Autodesk Inventor part; units mm, degrees
(part 2 of 4)
  line L557 (-1.0373, -25.9013) -> (-0.4998, -25.9013)
  spline S119 degree 2 poles (-0.4998, -25.9013) (-0.366, -25.9013) (-0.366, -26.0351) knots 0 0 0 1 1 1
  line L558 (-0.4998, -25.9013) -> (-0.366, -25.9013) construction
  line L559 (-0.366, -25.9013) -> (-0.366, -26.0351) construction
  line L560 (-0.366, -26.0351) -> (-0.366, -27.6364)
  spline S120 degree 2 poles (-0.366, -27.6364) (-0.366, -27.7703) (-0.4998, -27.7703) knots 0 0 0 1 1 1
  line L561 (-0.366, -27.6364) -> (-0.366, -27.7703) construction
  line L562 (-0.366, -27.7703) -> (-0.4998, -27.7703) construction
  spline S121 degree 2 poles (-7.9758, -27.7703) (-8.1096, -27.7703) (-8.1096, -27.6364) knots 0 0 0 1 1 1
  line L563 (-7.9758, -27.7703) -> (-8.1096, -27.7703) construction
  line L564 (-8.1096, -27.7703) -> (-8.1096, -27.6364) construction
  line L565 (-8.1096, -27.6364) -> (-8.1096, -26.4365)
  spline S122 degree 2 poles (-8.1096, -26.4365) (-8.1096, -26.3273) (-8.2657, -26.1689) (-8.375, -26.1689) knots 0 0 0 1 2 2 2
  line L566 (-8.1096, -26.4365) -> (-8.1096, -26.3273) construction
  line L567 (-8.1096, -26.3273) -> (-8.2657, -26.1689) construction
  line L568 (-8.2657, -26.1689) -> (-8.375, -26.1689) construction
  spline S123 degree 2 poles (-8.908, -27.6364) (-8.908, -27.7703) (-9.0418, -27.7703) knots 0 0 0 1 1 1
  line L569 (-8.908, -27.6364) -> (-8.908, -27.7703) construction
  line L570 (-8.908, -27.7703) -> (-9.0418, -27.7703) construction
  spline S124 degree 2 poles (-9.0418, -27.7703) (-9.1756, -27.7703) (-9.1756, -27.6364) knots 0 0 0 1 1 1
  line L571 (-9.0418, -27.7703) -> (-9.1756, -27.7703) construction
  line L572 (-9.1756, -27.7703) -> (-9.1756, -27.6364) construction
  line L573 (-9.1756, -27.6364) -> (-9.1756, -26.0351)
  spline S125 degree 2 poles (-9.1756, -26.0351) (-9.1756, -25.9013) (-9.0418, -25.9013) knots 0 0 0 1 1 1
  line L574 (-9.1756, -26.0351) -> (-9.1756, -25.9013) construction
  line L575 (-9.1756, -25.9013) -> (-9.0418, -25.9013) construction
  line L576 (-9.0418, -25.9013) -> (-8.375, -25.9013)
  spline S126 degree 2 poles (-8.375, -25.9013) (-8.1542, -25.9013) (-7.8419, -26.2135) (-7.8419, -26.4343) knots 0 0 0 1 2 2 2
  line L577 (-8.375, -25.9013) -> (-8.1542, -25.9013) construction
  line L578 (-8.1542, -25.9013) -> (-7.8419, -26.2135) construction
  line L579 (-7.8419, -26.2135) -> (-7.8419, -26.4343) construction
  line L580 (-7.8419, -26.4343) -> (-7.8419, -27.6364)
  spline S127 degree 2 poles (-7.8419, -27.6364) (-7.8419, -27.7703) (-7.9758, -27.7703) knots 0 0 0 1 1 1
  line L581 (-7.8419, -27.6364) -> (-7.8419, -27.7703) construction
  line L582 (-7.8419, -27.7703) -> (-7.9758, -27.7703) construction
  spline S128 degree 2 poles (-10.2439, -27.5026) (-10.1347, -27.5026) (-9.9785, -27.3443) (-9.9785, -27.235) knots 0 0 0 1 2 2 2
  line L583 (-10.2439, -27.5026) -> (-10.1347, -27.5026) construction
  line L584 (-10.1347, -27.5026) -> (-9.9785, -27.3443) construction
  line L585 (-9.9785, -27.3443) -> (-9.9785, -27.235) construction
  spline S129 degree 2 poles (-10.5116, -26.1689) (-10.6209, -26.1689) (-10.777, -26.3273) (-10.777, -26.4365) knots 0 0 0 1 2 2 2
  line L586 (-10.5116, -26.1689) -> (-10.6209, -26.1689) construction
  line L587 (-10.6209, -26.1689) -> (-10.777, -26.3273) construction
  line L588 (-10.777, -26.3273) -> (-10.777, -26.4365) construction
  line L589 (-10.777, -26.4365) -> (-10.777, -27.235)
  spline S130 degree 2 poles (-10.777, -27.235) (-10.777, -27.3443) (-10.6209, -27.5026) (-10.5116, -27.5026) knots 0 0 0 1 2 2 2
  line L590 (-10.777, -27.235) -> (-10.777, -27.3443) construction
  line L591 (-10.777, -27.3443) -> (-10.6209, -27.5026) construction
  line L592 (-10.6209, -27.5026) -> (-10.5116, -27.5026) construction
  line L593 (-10.5116, -27.5026) -> (-10.2439, -27.5026)
  line L594 (-10.2439, -27.7703) -> (-10.5116, -27.7703)
  spline S131 degree 2 poles (-10.5116, -27.7703) (-10.7302, -27.7703) (-11.0446, -27.458) (-11.0446, -27.2372) knots 0 0 0 1 2 2 2
  line L595 (-10.5116, -27.7703) -> (-10.7302, -27.7703) construction
  line L596 (-10.7302, -27.7703) -> (-11.0446, -27.458) construction
  line L597 (-11.0446, -27.458) -> (-11.0446, -27.2372) construction
  line L598 (-11.0446, -27.2372) -> (-11.0446, -26.4343)
  spline S132 degree 2 poles (-11.0446, -26.4343) (-11.0446, -26.2135) (-10.7302, -25.9013) (-10.5116, -25.9013) knots 0 0 0 1 2 2 2
  line L599 (-11.0446, -26.4343) -> (-11.0446, -26.2135) construction
  line L600 (-11.0446, -26.2135) -> (-10.7302, -25.9013) construction
  line L601 (-10.7302, -25.9013) -> (-10.5116, -25.9013) construction
  line L602 (-10.5116, -25.9013) -> (-9.8447, -25.9013)
  spline S133 degree 2 poles (-9.8447, -25.9013) (-9.7109, -25.9013) (-9.7109, -26.0351) knots 0 0 0 1 1 1
  line L603 (-9.8447, -25.9013) -> (-9.7109, -25.9013) construction
  line L604 (-9.7109, -25.9013) -> (-9.7109, -26.0351) construction
  line L605 (-9.7109, -26.0351) -> (-9.7109, -27.2328)
  spline S134 degree 2 poles (-9.7109, -27.2328) (-9.7109, -27.4335) (-9.5236, -27.5138) knots 0 0 0 1 1 1
  line L606 (-9.7109, -27.2328) -> (-9.7109, -27.4335) construction
  line L607 (-9.7109, -27.4335) -> (-9.5236, -27.5138) construction
  spline S135 degree 2 poles (-9.5236, -27.5138) (-9.441, -27.5472) (-9.441, -27.632) knots 0 0 0 1 1 1
  line L608 (-9.5236, -27.5138) -> (-9.441, -27.5472) construction
  line L609 (-9.441, -27.5472) -> (-9.441, -27.632) construction
  spline S136 degree 2 poles (-9.441, -27.632) (-9.441, -27.6877) (-9.5169, -27.7725) (-9.5726, -27.7725) knots 0 0 0 1 2 2 2
  line L610 (-9.441, -27.632) -> (-9.441, -27.6877) construction
  line L611 (-9.441, -27.6877) -> (-9.5169, -27.7725) construction
  line L612 (-9.5169, -27.7725) -> (-9.5726, -27.7725) construction
  spline S137 degree 2 poles (-9.5726, -27.7725) (-9.6016, -27.7725) (-9.6306, -27.7591) knots 0 0 0 1 1 1
  line L613 (-9.5726, -27.7725) -> (-9.6016, -27.7725) construction
  line L614 (-9.6016, -27.7725) -> (-9.6306, -27.7591) construction
  spline S138 degree 2 poles (-9.6306, -27.7591) (-9.7644, -27.7011) (-9.847, -27.5941) knots 0 0 0 1 1 1
  line L615 (-9.6306, -27.7591) -> (-9.7644, -27.7011) construction
  line L616 (-9.7644, -27.7011) -> (-9.847, -27.5941) construction
  spline S139 degree 2 poles (-9.847, -27.5941) (-10.0075, -27.7703) (-10.2439, -27.7703) knots 0 0 0 1 1 1
  line L617 (-9.847, -27.5941) -> (-10.0075, -27.7703) construction
  line L618 (-10.0075, -27.7703) -> (-10.2439, -27.7703) construction
  spline S140 degree 2 poles (8.3441, 56.8614) (8.338, 56.6518) (8.3229, 56.2658) (8.3137, 56.1108) knots 0 0 0 1 2 2 2
  line L619 (8.3441, 56.8614) -> (8.338, 56.6518) construction
  line L620 (8.338, 56.6518) -> (8.3229, 56.2658) construction
  line L621 (8.3229, 56.2658) -> (8.3137, 56.1108) construction
  spline S141 degree 2 poles (8.3137, 56.1108) (8.2985, 55.7158) (8.2256, 55.1809) (8.1709, 55.0199) knots 0 0 0 1 2 2 2
  line L622 (8.3137, 56.1108) -> (8.2985, 55.7158) construction
  line L623 (8.2985, 55.7158) -> (8.2256, 55.1809) construction
  line L624 (8.2256, 55.1809) -> (8.1709, 55.0199) construction
  spline S142 degree 2 poles (8.1709, 55.0199) (8.1162, 54.8527) (7.9825, 54.6674) (7.8974, 54.5914) knots 0 0 0 1 2 2 2
  line L625 (8.1709, 55.0199) -> (8.1162, 54.8527) construction
  line L626 (8.1162, 54.8527) -> (7.9825, 54.6674) construction
  line L627 (7.9825, 54.6674) -> (7.8974, 54.5914) construction
  spline S143 degree 2 poles (7.8974, 54.5914) (7.8123, 54.5154) (7.6178, 54.4394) (7.4932, 54.4394) knots 0 0 0 1 2 2 2
  line L628 (7.8974, 54.5914) -> (7.8123, 54.5154) construction
  line L629 (7.8123, 54.5154) -> (7.6178, 54.4394) construction
  line L630 (7.6178, 54.4394) -> (7.4932, 54.4394) construction
  spline S144 degree 2 poles (7.4932, 54.4394) (7.4537, 54.4394) (7.3261, 54.4455) (7.3018, 54.4455) knots 0 0 0 1 2 2 2
  line L631 (7.4932, 54.4394) -> (7.4537, 54.4394) construction
  line L632 (7.4537, 54.4394) -> (7.3261, 54.4455) construction
  line L633 (7.3261, 54.4455) -> (7.3018, 54.4455) construction
  spline S145 degree 2 poles (7.3261, 54.8588) (7.3443, 54.8588) (7.3838, 54.8527) (7.4081, 54.8527) knots 0 0 0 1 2 2 2
  line L634 (7.3261, 54.8588) -> (7.3443, 54.8588) construction
  line L635 (7.3443, 54.8588) -> (7.3838, 54.8527) construction
  line L636 (7.3838, 54.8527) -> (7.4081, 54.8527) construction
  spline S146 degree 2 poles (7.4081, 54.8527) (7.4689, 54.8527) (7.5844, 54.8892) (7.63, 54.9348) knots 0 0 0 1 2 2 2
  line L637 (7.4081, 54.8527) -> (7.4689, 54.8527) construction
  line L638 (7.4689, 54.8527) -> (7.5844, 54.8892) construction
  line L639 (7.5844, 54.8892) -> (7.63, 54.9348) construction
  spline S147 degree 2 poles (7.63, 54.9348) (7.7546, 55.0594) (7.8701, 55.6763) (7.8944, 56.2324) knots 0 0 0 1 2 2 2
  line L640 (7.63, 54.9348) -> (7.7546, 55.0594) construction
  line L641 (7.7546, 55.0594) -> (7.8701, 55.6763) construction
  line L642 (7.8701, 55.6763) -> (7.8944, 56.2324) construction
  spline S148 degree 2 poles (7.8944, 56.2324) (7.9065, 56.439) (7.9248, 57.0012) (7.9308, 57.2595) knots 0 0 0 1 2 2 2
  line L643 (7.8944, 56.2324) -> (7.9065, 56.439) construction
  line L644 (7.9065, 56.439) -> (7.9248, 57.0012) construction
  line L645 (7.9248, 57.0012) -> (7.9308, 57.2595) construction
  spline S149 degree 2 poles (5.8674, 54.7737) (6.2321, 54.7737) (6.6332, 55.3116) (6.6332, 55.8525) knots 0 0 0 1 2 2 2
  line L646 (5.8674, 54.7737) -> (6.2321, 54.7737) construction
  line L647 (6.2321, 54.7737) -> (6.6332, 55.3116) construction
  line L648 (6.6332, 55.3116) -> (6.6332, 55.8525) construction
  spline S150 degree 2 poles (6.6332, 55.8525) (6.6332, 56.3995) (6.2351, 56.9313) (5.8674, 56.9313) knots 0 0 0 1 2 2 2
  line L649 (6.6332, 55.8525) -> (6.6332, 56.3995) construction
  line L650 (6.6332, 56.3995) -> (6.2351, 56.9313) construction
  line L651 (6.2351, 56.9313) -> (5.8674, 56.9313) construction
  spline S151 degree 2 poles (5.8674, 56.9313) (5.4997, 56.9313) (5.0986, 56.3995) (5.0986, 55.8525) knots 0 0 0 1 2 2 2
  line L652 (5.8674, 56.9313) -> (5.4997, 56.9313) construction
  line L653 (5.4997, 56.9313) -> (5.0986, 56.3995) construction
  line L654 (5.0986, 56.3995) -> (5.0986, 55.8525) construction
  spline S152 degree 2 poles (5.0986, 55.8525) (5.0986, 55.3207) (5.4997, 54.7737) (5.8674, 54.7737) knots 0 0 0 1 2 2 2
  line L655 (5.0986, 55.8525) -> (5.0986, 55.3207) construction
  line L656 (5.0986, 55.3207) -> (5.4997, 54.7737) construction
  line L657 (5.4997, 54.7737) -> (5.8674, 54.7737) construction
  spline S153 degree 2 poles (5.8674, 54.3665) (5.2809, 54.3665) (4.6093, 55.1657) (4.6093, 55.8525) knots 0 0 0 1 2 2 2
  line L658 (5.8674, 54.3665) -> (5.2809, 54.3665) construction
  line L659 (5.2809, 54.3665) -> (4.6093, 55.1657) construction
  line L660 (4.6093, 55.1657) -> (4.6093, 55.8525) construction
  spline S154 degree 2 poles (4.6093, 55.8525) (4.6093, 56.5575) (5.3022, 57.3385) (5.8674, 57.3385) knots 0 0 0 1 2 2 2
  line L661 (4.6093, 55.8525) -> (4.6093, 56.5575) construction
  line L662 (4.6093, 56.5575) -> (5.3022, 57.3385) construction
  line L663 (5.3022, 57.3385) -> (5.8674, 57.3385) construction
  spline S155 degree 2 poles (5.8674, 57.3385) (6.4387, 57.3385) (7.1225, 56.5606) (7.1225, 55.8525) knots 0 0 0 1 2 2 2
  line L664 (5.8674, 57.3385) -> (6.4387, 57.3385) construction
  line L665 (6.4387, 57.3385) -> (7.1225, 56.5606) construction
  line L666 (7.1225, 56.5606) -> (7.1225, 55.8525) construction
  spline S156 degree 2 poles (7.1225, 55.8525) (7.1225, 55.1414) (6.4387, 54.3665) (5.8674, 54.3665) knots 0 0 0 1 2 2 2
  line L667 (7.1225, 55.8525) -> (7.1225, 55.1414) construction
  line L668 (7.1225, 55.1414) -> (6.4387, 54.3665) construction
  line L669 (6.4387, 54.3665) -> (5.8674, 54.3665) construction
  spline S157 degree 2 poles (3.0534, 54.8163) (3.4211, 54.8163) (3.8283, 55.3572) (3.8283, 55.8738) knots 0 0 0 1 2 2 2
  line L670 (3.0534, 54.8163) -> (3.4211, 54.8163) construction
  line L671 (3.4211, 54.8163) -> (3.8283, 55.3572) construction
  line L672 (3.8283, 55.3572) -> (3.8283, 55.8738) construction
  spline S158 degree 2 poles (3.8283, 55.8738) (3.8283, 56.357) (3.5214, 56.8888) (3.178, 56.8888) knots 0 0 0 1 2 2 2
  line L673 (3.8283, 55.8738) -> (3.8283, 56.357) construction
  line L674 (3.8283, 56.357) -> (3.5214, 56.8888) construction
  line L675 (3.5214, 56.8888) -> (3.178, 56.8888) construction
  spline S159 degree 2 poles (3.178, 56.8888) (2.9774, 56.8888) (2.6006, 56.7095) (2.4335, 56.5697) knots 0 0 0 1 2 2 2
  line L676 (3.178, 56.8888) -> (2.9774, 56.8888) construction
  line L677 (2.9774, 56.8888) -> (2.6006, 56.7095) construction
  line L678 (2.6006, 56.7095) -> (2.4335, 56.5697) construction
  line L679 (2.4335, 56.5697) -> (2.4335, 54.9712)
  spline S160 degree 2 poles (2.4335, 54.9712) (2.6188, 54.8831) (2.8832, 54.8163) (3.0534, 54.8163) knots 0 0 0 1 2 2 2
  line L680 (2.4335, 54.9712) -> (2.6188, 54.8831) construction
  line L681 (2.6188, 54.8831) -> (2.8832, 54.8163) construction
  line L682 (2.8832, 54.8163) -> (3.0534, 54.8163) construction
  spline S161 degree 2 poles (3.1324, 54.3908) (2.9227, 54.3908) (2.6006, 54.4881) (2.4335, 54.5883) knots 0 0 0 1 2 2 2
  line L683 (3.1324, 54.3908) -> (2.9227, 54.3908) construction
  line L684 (2.9227, 54.3908) -> (2.6006, 54.4881) construction
  line L685 (2.6006, 54.4881) -> (2.4335, 54.5883) construction
  spline S162 degree 2 poles (2.4335, 56.9648) (2.6097, 57.1258) (3.0412, 57.3385) (3.2935, 57.3385) knots 0 0 0 1 2 2 2
  line L686 (2.4335, 56.9648) -> (2.6097, 57.1258) construction
  line L687 (2.6097, 57.1258) -> (3.0412, 57.3385) construction
  line L688 (3.0412, 57.3385) -> (3.2935, 57.3385) construction
  spline S163 degree 2 poles (3.2935, 57.3385) (3.7767, 57.3385) (4.3176, 56.5727) (4.3176, 55.9285) knots 0 0 0 1 2 2 2
  line L689 (3.2935, 57.3385) -> (3.7767, 57.3385) construction
  line L690 (3.7767, 57.3385) -> (4.3176, 56.5727) construction
  line L691 (4.3176, 56.5727) -> (4.3176, 55.9285) construction
  spline S164 degree 2 poles (4.3176, 55.9285) (4.3176, 55.2235) (3.646, 54.3908) (3.1324, 54.3908) knots 0 0 0 1 2 2 2
  line L692 (4.3176, 55.9285) -> (4.3176, 55.2235) construction
  line L693 (4.3176, 55.2235) -> (3.646, 54.3908) construction
  line L694 (3.646, 54.3908) -> (3.1324, 54.3908) construction
  spline S165 degree 2 poles (-5.0908, 54.7737) (-4.7262, 54.7737) (-4.325, 55.3116) (-4.325, 55.8525) knots 0 0 0 1 2 2 2
  line L695 (-5.0908, 54.7737) -> (-4.7262, 54.7737) construction
  line L696 (-4.7262, 54.7737) -> (-4.325, 55.3116) construction
  line L697 (-4.325, 55.3116) -> (-4.325, 55.8525) construction
  spline S166 degree 2 poles (-4.325, 55.8525) (-4.325, 56.3995) (-4.7231, 56.9313) (-5.0908, 56.9313) knots 0 0 0 1 2 2 2
  line L698 (-4.325, 55.8525) -> (-4.325, 56.3995) construction
  line L699 (-4.325, 56.3995) -> (-4.7231, 56.9313) construction
  line L700 (-4.7231, 56.9313) -> (-5.0908, 56.9313) construction
  spline S167 degree 2 poles (-5.0908, 56.9313) (-5.4585, 56.9313) (-5.8597, 56.3995) (-5.8597, 55.8525) knots 0 0 0 1 2 2 2
  line L701 (-5.0908, 56.9313) -> (-5.4585, 56.9313) construction
  line L702 (-5.4585, 56.9313) -> (-5.8597, 56.3995) construction
  line L703 (-5.8597, 56.3995) -> (-5.8597, 55.8525) construction
  spline S168 degree 2 poles (-5.8597, 55.8525) (-5.8597, 55.3207) (-5.4585, 54.7737) (-5.0908, 54.7737) knots 0 0 0 1 2 2 2
  line L704 (-5.8597, 55.8525) -> (-5.8597, 55.3207) construction
  line L705 (-5.8597, 55.3207) -> (-5.4585, 54.7737) construction
  line L706 (-5.4585, 54.7737) -> (-5.0908, 54.7737) construction
  spline S169 degree 2 poles (-5.0908, 54.3665) (-5.6773, 54.3665) (-6.3489, 55.1657) (-6.3489, 55.8525) knots 0 0 0 1 2 2 2
  line L707 (-5.0908, 54.3665) -> (-5.6773, 54.3665) construction
  line L708 (-5.6773, 54.3665) -> (-6.3489, 55.1657) construction
  line L709 (-6.3489, 55.1657) -> (-6.3489, 55.8525) construction
  spline S170 degree 2 poles (-6.3489, 55.8525) (-6.3489, 56.5575) (-5.6561, 57.3385) (-5.0908, 57.3385) knots 0 0 0 1 2 2 2
  line L710 (-6.3489, 55.8525) -> (-6.3489, 56.5575) construction
  line L711 (-6.3489, 56.5575) -> (-5.6561, 57.3385) construction
  line L712 (-5.6561, 57.3385) -> (-5.0908, 57.3385) construction
  spline S171 degree 2 poles (-5.0908, 57.3385) (-4.5195, 57.3385) (-3.8358, 56.5606) (-3.8358, 55.8525) knots 0 0 0 1 2 2 2
  line L713 (-5.0908, 57.3385) -> (-4.5195, 57.3385) construction
  line L714 (-4.5195, 57.3385) -> (-3.8358, 56.5606) construction
  line L715 (-3.8358, 56.5606) -> (-3.8358, 55.8525) construction
  spline S172 degree 2 poles (-3.8358, 55.8525) (-3.8358, 55.1414) (-4.5195, 54.3665) (-5.0908, 54.3665) knots 0 0 0 1 2 2 2
  line L716 (-3.8358, 55.8525) -> (-3.8358, 55.1414) construction
  line L717 (-3.8358, 55.1414) -> (-4.5195, 54.3665) construction
  line L718 (-4.5195, 54.3665) -> (-5.0908, 54.3665) construction
  spline S173 degree 2 poles (-1.0482, 51.3101) (-0.9233, 51.3101) (-0.8497, 51.3926) knots 0 0 0 1 1 1
  line L719 (-1.0482, 51.3101) -> (-0.9233, 51.3101) construction
  line L720 (-0.9233, 51.3101) -> (-0.8497, 51.3926) construction
  spline S174 degree 2 poles (-0.8497, 51.3926) (-0.7828, 51.4684) (-0.7828, 51.5777) knots 0 0 0 1 1 1
  line L721 (-0.8497, 51.3926) -> (-0.7828, 51.4684) construction
  line L722 (-0.7828, 51.4684) -> (-0.7828, 51.5777) construction
  spline S175 degree 2 poles (-0.7828, 51.5777) (-0.7828, 51.687) (-0.8497, 51.7606) knots 0 0 0 1 1 1
  line L723 (-0.7828, 51.5777) -> (-0.7828, 51.687) construction
  line L724 (-0.7828, 51.687) -> (-0.8497, 51.7606) construction
  spline S176 degree 2 poles (-0.8497, 51.7606) (-0.9233, 51.8431) (-1.0482, 51.8431) knots 0 0 0 1 1 1
  line L725 (-0.8497, 51.7606) -> (-0.9233, 51.8431) construction
  line L726 (-0.9233, 51.8431) -> (-1.0482, 51.8431) construction
  spline S177 degree 2 poles (-1.0482, 52.1107) (-0.7962, 52.1107) (-0.649, 51.9435) knots 0 0 0 1 1 1
  line L727 (-1.0482, 52.1107) -> (-0.7962, 52.1107) construction
  line L728 (-0.7962, 52.1107) -> (-0.649, 51.9435) construction
  spline S178 degree 2 poles (-0.649, 51.9435) (-0.5152, 51.794) (-0.5152, 51.5777) knots 0 0 0 1 1 1
  line L729 (-0.649, 51.9435) -> (-0.5152, 51.794) construction
  line L730 (-0.5152, 51.794) -> (-0.5152, 51.5777) construction
  spline S179 degree 2 poles (-0.5152, 51.5777) (-0.5152, 51.3614) (-0.649, 51.2075) knots 0 0 0 1 1 1
  line L731 (-0.5152, 51.5777) -> (-0.5152, 51.3614) construction
  line L732 (-0.5152, 51.3614) -> (-0.649, 51.2075) construction
  spline S180 degree 2 poles (-0.649, 51.2075) (-0.7962, 51.0424) (-1.0482, 51.0424) knots 0 0 0 1 1 1
  line L733 (-0.649, 51.2075) -> (-0.7962, 51.0424) construction
  line L734 (-0.7962, 51.0424) -> (-1.0482, 51.0424) construction
  line L735 (-1.0482, 51.0424) -> (-1.4496, 51.0424)
  spline S181 degree 2 poles (-1.4496, 51.0424) (-1.5835, 51.0424) (-1.5835, 51.1763) knots 0 0 0 1 1 1
  line L736 (-1.4496, 51.0424) -> (-1.5835, 51.0424) construction
  line L737 (-1.5835, 51.0424) -> (-1.5835, 51.1763) construction
  line L738 (-1.5835, 51.1763) -> (-1.5835, 52.7776)
  spline S182 degree 2 poles (-1.5835, 52.7776) (-1.5835, 52.9114) (-1.4496, 52.9114) knots 0 0 0 1 1 1
  line L739 (-1.5835, 52.7776) -> (-1.5835, 52.9114) construction
  line L740 (-1.5835, 52.9114) -> (-1.4496, 52.9114) construction
  spline S183 degree 2 poles (-1.4496, 52.9114) (-1.3158, 52.9114) (-1.3158, 52.7776) knots 0 0 0 1 1 1
  line L741 (-1.4496, 52.9114) -> (-1.3158, 52.9114) construction
  line L742 (-1.3158, 52.9114) -> (-1.3158, 52.7776) construction
  spline S184 degree 2 poles (-7.7257, 51.1763) (-7.7257, 51.0424) (-7.8595, 51.0424) knots 0 0 0 1 1 1
  line L743 (-7.7257, 51.1763) -> (-7.7257, 51.0424) construction
  line L744 (-7.7257, 51.0424) -> (-7.8595, 51.0424) construction
  spline S185 degree 2 poles (-7.8595, 51.0424) (-7.9933, 51.0424) (-7.9933, 51.1763) knots 0 0 0 1 1 1
  line L745 (-7.8595, 51.0424) -> (-7.9933, 51.0424) construction
  line L746 (-7.9933, 51.0424) -> (-7.9933, 51.1763) construction
  line L747 (-7.9933, 51.1763) -> (-7.9933, 52.7776)
  spline S186 degree 2 poles (-7.9933, 52.7776) (-7.9933, 52.9114) (-7.8595, 52.9114) knots 0 0 0 1 1 1
  line L748 (-7.9933, 52.7776) -> (-7.9933, 52.9114) construction
  line L749 (-7.9933, 52.9114) -> (-7.8595, 52.9114) construction
  line L750 (-7.8595, 52.9114) -> (-6.6574, 52.9114)
  spline S187 degree 2 poles (-6.6574, 52.9114) (-6.4366, 52.9114) (-6.1243, 52.5992) (-6.1243, 52.3784) knots 0 0 0 1 2 2 2
  line L751 (-6.6574, 52.9114) -> (-6.4366, 52.9114) construction
  line L752 (-6.4366, 52.9114) -> (-6.1243, 52.5992) construction
  line L753 (-6.1243, 52.5992) -> (-6.1243, 52.3784) construction
  line L754 (-6.1243, 52.3784) -> (-6.1243, 51.1763)
  spline S188 degree 2 poles (-6.1243, 51.1763) (-6.1243, 51.0424) (-6.2581, 51.0424) knots 0 0 0 1 1 1
  line L755 (-6.1243, 51.1763) -> (-6.1243, 51.0424) construction
  line L756 (-6.1243, 51.0424) -> (-6.2581, 51.0424) construction
  spline S189 degree 2 poles (-6.2581, 51.0424) (-6.392, 51.0424) (-6.392, 51.1763) knots 0 0 0 1 1 1
  line L757 (-6.2581, 51.0424) -> (-6.392, 51.0424) construction
  line L758 (-6.392, 51.0424) -> (-6.392, 51.1763) construction
  line L759 (-6.392, 51.1763) -> (-6.392, 52.3762)
  spline S190 degree 2 poles (-6.392, 52.3762) (-6.392, 52.4854) (-6.5481, 52.6438) (-6.6574, 52.6438) knots 0 0 0 1 2 2 2
  line L760 (-6.392, 52.3762) -> (-6.392, 52.4854) construction
  line L761 (-6.392, 52.4854) -> (-6.5481, 52.6438) construction
  line L762 (-6.5481, 52.6438) -> (-6.6574, 52.6438) construction
  spline S191 degree 2 poles (-6.925, 51.1763) (-6.925, 51.0424) (-7.0588, 51.0424) knots 0 0 0 1 1 1
  line L763 (-6.925, 51.1763) -> (-6.925, 51.0424) construction
  line L764 (-6.925, 51.0424) -> (-7.0588, 51.0424) construction
  spline S192 degree 2 poles (-7.0588, 51.0424) (-7.1926, 51.0424) (-7.1926, 51.1763) knots 0 0 0 1 1 1
  line L765 (-7.0588, 51.0424) -> (-7.1926, 51.0424) construction
  line L766 (-7.1926, 51.0424) -> (-7.1926, 51.1763) construction
  line L767 (-10.2637, 51.0424) -> (-10.9306, 51.0424)
  spline S193 degree 2 poles (-10.9306, 51.0424) (-11.1492, 51.0424) (-11.4636, 51.3547) (-11.4636, 51.5755) knots 0 0 0 1 2 2 2
  line L768 (-10.9306, 51.0424) -> (-11.1492, 51.0424) construction
  line L769 (-11.1492, 51.0424) -> (-11.4636, 51.3547) construction
  line L770 (-11.4636, 51.3547) -> (-11.4636, 51.5755) construction
  line L771 (-11.4636, 51.5755) -> (-11.4636, 52.7776)
  spline S194 degree 2 poles (-11.4636, 52.7776) (-11.4636, 52.9114) (-11.3298, 52.9114) knots 0 0 0 1 1 1
  line L772 (-11.4636, 52.7776) -> (-11.4636, 52.9114) construction
  line L773 (-11.4636, 52.9114) -> (-11.3298, 52.9114) construction
  spline S195 degree 2 poles (-11.3298, 52.9114) (-11.196, 52.9114) (-11.196, 52.7776) knots 0 0 0 1 1 1
  line L774 (-11.3298, 52.9114) -> (-11.196, 52.9114) construction
  line L775 (-11.196, 52.9114) -> (-11.196, 52.7776) construction
  line L776 (-11.196, 52.7776) -> (-11.196, 51.5777)
  spline S196 degree 2 poles (-11.196, 51.5777) (-11.196, 51.4684) (-11.0399, 51.3101) (-10.9306, 51.3101) knots 0 0 0 1 2 2 2
  line L777 (-11.196, 51.5777) -> (-11.196, 51.4684) construction
  line L778 (-11.196, 51.4684) -> (-11.0399, 51.3101) construction
  line L779 (-11.0399, 51.3101) -> (-10.9306, 51.3101) construction
  spline S197 degree 2 poles (-10.3975, 52.7776) (-10.3975, 52.9114) (-10.2637, 52.9114) knots 0 0 0 1 1 1
  line L780 (-10.3975, 52.7776) -> (-10.3975, 52.9114) construction
  line L781 (-10.3975, 52.9114) -> (-10.2637, 52.9114) construction
  spline S198 degree 2 poles (-10.2637, 52.9114) (-10.1299, 52.9114) (-10.1299, 52.7776) knots 0 0 0 1 1 1
  line L782 (-10.2637, 52.9114) -> (-10.1299, 52.9114) construction
  line L783 (-10.1299, 52.9114) -> (-10.1299, 52.7776) construction
  line L784 (-10.1299, 52.7776) -> (-10.1299, 51.1763)
  spline S199 degree 2 poles (-10.1299, 51.1763) (-10.1299, 51.0424) (-10.2637, 51.0424) knots 0 0 0 1 1 1
  line L785 (-10.1299, 51.1763) -> (-10.1299, 51.0424) construction
  line L786 (-10.1299, 51.0424) -> (-10.2637, 51.0424) construction
  circle A32 centre (0.0461, -47.8325) radius 6.0897
  circle A33 centre (0.0461, -47.8325) radius 6.6254
  spline S200 degree 2 poles (-12.5297, 51.0424) (-12.7483, 51.0424) (-13.065, 51.3547) (-13.065, 51.5755) knots 0 0 0 1 2 2 2
  line L787 (-12.5297, 51.0424) -> (-12.7483, 51.0424) construction
  line L788 (-12.7483, 51.0424) -> (-13.065, 51.3547) construction
  line L789 (-13.065, 51.3547) -> (-13.065, 51.5755) construction
  line L790 (-13.065, 51.5755) -> (-13.065, 52.3784)
  spline S201 degree 2 poles (-13.065, 52.3784) (-13.065, 52.5992) (-12.7483, 52.9114) (-12.5297, 52.9114) knots 0 0 0 1 2 2 2
  line L791 (-13.065, 52.3784) -> (-13.065, 52.5992) construction
  line L792 (-13.065, 52.5992) -> (-12.7483, 52.9114) construction
  line L793 (-12.7483, 52.9114) -> (-12.5297, 52.9114) construction
  line L794 (-12.5297, 52.9114) -> (-12.1305, 52.9114)
  spline S202 degree 2 poles (-12.1305, 52.9114) (-11.9967, 52.9114) (-11.9967, 52.7776) knots 0 0 0 1 1 1
  line L795 (-12.1305, 52.9114) -> (-11.9967, 52.9114) construction
  line L796 (-11.9967, 52.9114) -> (-11.9967, 52.7776) construction
  spline S203 degree 2 poles (-11.9967, 52.7776) (-11.9967, 52.6438) (-12.1305, 52.6438) knots 0 0 0 1 1 1
  line L797 (-11.9967, 52.7776) -> (-11.9967, 52.6438) construction
  line L798 (-11.9967, 52.6438) -> (-12.1305, 52.6438) construction
  line L799 (-12.1305, 52.6438) -> (-12.5297, 52.6438)
  spline S204 degree 2 poles (-12.5297, 52.6438) (-12.639, 52.6438) (-12.7973, 52.4854) (-12.7973, 52.3762) knots 0 0 0 1 2 2 2
  line L800 (-12.5297, 52.6438) -> (-12.639, 52.6438) construction
  line L801 (-12.639, 52.6438) -> (-12.7973, 52.4854) construction
  line L802 (-12.7973, 52.4854) -> (-12.7973, 52.3762) construction
  line L803 (-12.7973, 52.3762) -> (-12.7973, 51.5777)
  spline S205 degree 2 poles (-12.7973, 51.5777) (-12.7973, 51.4684) (-12.639, 51.3101) (-12.5297, 51.3101) knots 0 0 0 1 2 2 2
  line L804 (-12.7973, 51.5777) -> (-12.7973, 51.4684) construction
  line L805 (-12.7973, 51.4684) -> (-12.639, 51.3101) construction
  line L806 (-12.639, 51.3101) -> (-12.5297, 51.3101) construction
  line L807 (-12.5297, 51.3101) -> (-12.1305, 51.3101)
  spline S206 degree 2 poles (-12.1305, 51.3101) (-11.9967, 51.3101) (-11.9967, 51.1763) knots 0 0 0 1 1 1
  line L808 (-12.1305, 51.3101) -> (-11.9967, 51.3101) construction
  line L809 (-11.9967, 51.3101) -> (-11.9967, 51.1763) construction
  spline S207 degree 2 poles (-11.9967, 51.1763) (-11.9967, 51.0424) (-12.1305, 51.0424) knots 0 0 0 1 1 1
  line L810 (-11.9967, 51.1763) -> (-11.9967, 51.0424) construction
  line L811 (-11.9967, 51.0424) -> (-12.1305, 51.0424) construction
  line L812 (-12.1305, 51.0424) -> (-12.5297, 51.0424)
  spline S208 degree 2 poles (-9.0594, 51.0424) (-9.2779, 51.0424) (-9.5946, 51.3547) (-9.5946, 51.5755) knots 0 0 0 1 2 2 2
  line L813 (-9.0594, 51.0424) -> (-9.2779, 51.0424) construction
  line L814 (-9.2779, 51.0424) -> (-9.5946, 51.3547) construction
  line L815 (-9.5946, 51.3547) -> (-9.5946, 51.5755) construction
  line L816 (-9.5946, 51.5755) -> (-9.5946, 52.3784)
  spline S209 degree 2 poles (-9.5946, 52.3784) (-9.5946, 52.5992) (-9.2779, 52.9114) (-9.0594, 52.9114) knots 0 0 0 1 2 2 2
  line L817 (-9.5946, 52.3784) -> (-9.5946, 52.5992) construction
  line L818 (-9.5946, 52.5992) -> (-9.2779, 52.9114) construction
  line L819 (-9.2779, 52.9114) -> (-9.0594, 52.9114) construction
  line L820 (-9.0594, 52.9114) -> (-8.6602, 52.9114)
  spline S210 degree 2 poles (-8.6602, 52.9114) (-8.5263, 52.9114) (-8.5263, 52.7776) knots 0 0 0 1 1 1
  line L821 (-8.6602, 52.9114) -> (-8.5263, 52.9114) construction
  line L822 (-8.5263, 52.9114) -> (-8.5263, 52.7776) construction
  spline S211 degree 2 poles (-8.5263, 52.7776) (-8.5263, 52.6438) (-8.6602, 52.6438) knots 0 0 0 1 1 1
  line L823 (-8.5263, 52.7776) -> (-8.5263, 52.6438) construction
  line L824 (-8.5263, 52.6438) -> (-8.6602, 52.6438) construction
  line L825 (-8.6602, 52.6438) -> (-9.0594, 52.6438)
  spline S212 degree 2 poles (-9.0594, 52.6438) (-9.1687, 52.6438) (-9.327, 52.4854) (-9.327, 52.3762) knots 0 0 0 1 2 2 2
  line L826 (-9.0594, 52.6438) -> (-9.1687, 52.6438) construction
  line L827 (-9.1687, 52.6438) -> (-9.327, 52.4854) construction
  line L828 (-9.327, 52.4854) -> (-9.327, 52.3762) construction
  line L829 (-9.327, 52.3762) -> (-9.327, 51.5777)
  spline S213 degree 2 poles (-9.327, 51.5777) (-9.327, 51.4684) (-9.1687, 51.3101) (-9.0594, 51.3101) knots 0 0 0 1 2 2 2
  line L830 (-9.327, 51.5777) -> (-9.327, 51.4684) construction
  line L831 (-9.327, 51.4684) -> (-9.1687, 51.3101) construction
  line L832 (-9.1687, 51.3101) -> (-9.0594, 51.3101) construction
  line L833 (-9.0594, 51.3101) -> (-8.6602, 51.3101)
  spline S214 degree 2 poles (-8.6602, 51.3101) (-8.5263, 51.3101) (-8.5263, 51.1763) knots 0 0 0 1 1 1
  line L834 (-8.6602, 51.3101) -> (-8.5263, 51.3101) construction
  line L835 (-8.5263, 51.3101) -> (-8.5263, 51.1763) construction
  spline S215 degree 2 poles (-8.5263, 51.1763) (-8.5263, 51.0424) (-8.6602, 51.0424) knots 0 0 0 1 1 1
  line L836 (-8.5263, 51.1763) -> (-8.5263, 51.0424) construction
  line L837 (-8.5263, 51.0424) -> (-8.6602, 51.0424) construction
  line L838 (-8.6602, 51.0424) -> (-9.0594, 51.0424)
  spline S216 degree 2 poles (-4.523, 52.3784) (-4.523, 52.4877) (-4.6791, 52.6438) (-4.7884, 52.6438) knots 0 0 0 1 2 2 2
  line L839 (-4.523, 52.3784) -> (-4.523, 52.4877) construction
  line L840 (-4.523, 52.4877) -> (-4.6791, 52.6438) construction
  line L841 (-4.6791, 52.6438) -> (-4.7884, 52.6438) construction
  line L842 (-4.7884, 52.6438) -> (-5.056, 52.6438)
  spline S217 degree 2 poles (-5.056, 52.6438) (-5.1653, 52.6438) (-5.3214, 52.4877) (-5.3214, 52.3784) knots 0 0 0 1 2 2 2
  line L843 (-5.056, 52.6438) -> (-5.1653, 52.6438) construction
  line L844 (-5.1653, 52.6438) -> (-5.3214, 52.4877) construction
  line L845 (-5.3214, 52.4877) -> (-5.3214, 52.3784) construction
  spline S218 degree 2 poles (-5.3214, 51.5777) (-5.3214, 51.4684) (-5.1631, 51.3101) (-5.0538, 51.3101) knots 0 0 0 1 2 2 2
  line L846 (-5.3214, 51.5777) -> (-5.3214, 51.4684) construction
  line L847 (-5.3214, 51.4684) -> (-5.1631, 51.3101) construction
  line L848 (-5.1631, 51.3101) -> (-5.0538, 51.3101) construction
  line L849 (-5.0538, 51.3101) -> (-4.3892, 51.3101)
  spline S219 degree 2 poles (-4.3892, 51.3101) (-4.2553, 51.3101) (-4.2553, 51.1763) knots 0 0 0 1 1 1
  line L850 (-4.3892, 51.3101) -> (-4.2553, 51.3101) construction
  line L851 (-4.2553, 51.3101) -> (-4.2553, 51.1763) construction
  spline S220 degree 2 poles (-4.2553, 51.1763) (-4.2553, 51.0424) (-4.3892, 51.0424) knots 0 0 0 1 1 1
  line L852 (-4.2553, 51.1763) -> (-4.2553, 51.0424) construction
  line L853 (-4.2553, 51.0424) -> (-4.3892, 51.0424) construction
  line L854 (-4.3892, 51.0424) -> (-5.056, 51.0424)
  spline S221 degree 2 poles (-5.056, 51.0424) (-5.2768, 51.0424) (-5.5891, 51.3547) (-5.5891, 51.5755) knots 0 0 0 1 2 2 2
  line L855 (-5.056, 51.0424) -> (-5.2768, 51.0424) construction
  line L856 (-5.2768, 51.0424) -> (-5.5891, 51.3547) construction
  line L857 (-5.5891, 51.3547) -> (-5.5891, 51.5755) construction
  line L858 (-5.5891, 51.5755) -> (-5.5891, 52.3784)
  spline S222 degree 2 poles (-5.5891, 52.3784) (-5.5891, 52.5992) (-5.2768, 52.9114) (-5.056, 52.9114) knots 0 0 0 1 2 2 2
  line L859 (-5.5891, 52.3784) -> (-5.5891, 52.5992) construction
  line L860 (-5.5891, 52.5992) -> (-5.2768, 52.9114) construction
  line L861 (-5.2768, 52.9114) -> (-5.056, 52.9114) construction
  line L862 (-5.056, 52.9114) -> (-4.7884, 52.9114)
  spline S223 degree 2 poles (-4.7884, 52.9114) (-4.5676, 52.9114) (-4.2553, 52.5992) (-4.2553, 52.3784) knots 0 0 0 1 2 2 2
  line L863 (-4.7884, 52.9114) -> (-4.5676, 52.9114) construction
  line L864 (-4.5676, 52.9114) -> (-4.2553, 52.5992) construction
  line L865 (-4.2553, 52.5992) -> (-4.2553, 52.3784) construction
  line L866 (-4.2553, 52.3784) -> (-4.2553, 51.9769)
  spline S224 degree 2 poles (-4.2553, 51.9769) (-4.2553, 51.8431) (-4.3892, 51.8431) knots 0 0 0 1 1 1
  line L867 (-4.2553, 51.9769) -> (-4.2553, 51.8431) construction
  line L868 (-4.2553, 51.8431) -> (-4.3892, 51.8431) construction
  spline S225 degree 2 poles (-2.2525, 51.0424) (-2.3864, 51.0424) (-2.3864, 51.1763) knots 0 0 0 1 1 1
  line L869 (-2.2525, 51.0424) -> (-2.3864, 51.0424) construction
  line L870 (-2.3864, 51.0424) -> (-2.3864, 51.1763) construction
  spline S226 degree 2 poles (-2.8101, 51.7673) (-2.8614, 51.6937) (-2.9194, 51.6937) knots 0 0 0 1 1 1
  line L871 (-2.8101, 51.7673) -> (-2.8614, 51.6937) construction
  line L872 (-2.8614, 51.6937) -> (-2.9194, 51.6937) construction
  spline S227 degree 2 poles (-2.9194, 51.6937) (-2.9774, 51.6937) (-3.0287, 51.7673) knots 0 0 0 1 1 1
  line L873 (-2.9194, 51.6937) -> (-2.9774, 51.6937) construction
  line L874 (-2.9774, 51.6937) -> (-3.0287, 51.7673) construction
  spline S228 degree 2 poles (-3.4524, 51.1763) (-3.4524, 51.0424) (-3.5863, 51.0424) knots 0 0 0 1 1 1
  line L875 (-3.4524, 51.1763) -> (-3.4524, 51.0424) construction
  line L876 (-3.4524, 51.0424) -> (-3.5863, 51.0424) construction
  spline S229 degree 2 poles (-3.5863, 51.0424) (-3.7201, 51.0424) (-3.7201, 51.1763) knots 0 0 0 1 1 1
  line L877 (-3.5863, 51.0424) -> (-3.7201, 51.0424) construction
  line L878 (-3.7201, 51.0424) -> (-3.7201, 51.1763) construction
  line L879 (-3.7201, 51.1763) -> (-3.7201, 52.7798)
  spline S230 degree 2 poles (-3.7201, 52.7798) (-3.7201, 52.9337) (-3.6019, 52.9337) knots 0 0 0 1 1 1
  line L880 (-3.7201, 52.7798) -> (-3.7201, 52.9337) construction
  line L881 (-3.7201, 52.9337) -> (-3.6019, 52.9337) construction
  spline S231 degree 2 poles (-3.6019, 52.9337) (-3.5327, 52.9337) (-3.477, 52.8557) knots 0 0 0 1 1 1
  line L882 (-3.6019, 52.9337) -> (-3.5327, 52.9337) construction
  line L883 (-3.5327, 52.9337) -> (-3.477, 52.8557) construction
  spline S232 degree 2 poles (-2.3618, 52.8557) (-2.3061, 52.9337) (-2.2369, 52.9337) knots 0 0 0 1 1 1
  line L884 (-2.3618, 52.8557) -> (-2.3061, 52.9337) construction
  line L885 (-2.3061, 52.9337) -> (-2.2369, 52.9337) construction
  spline S233 degree 2 poles (-2.2369, 52.9337) (-2.1187, 52.9337) (-2.1187, 52.7798) knots 0 0 0 1 1 1
  line L886 (-2.2369, 52.9337) -> (-2.1187, 52.9337) construction
  line L887 (-2.1187, 52.9337) -> (-2.1187, 52.7798) construction
  line L888 (-2.1187, 52.7798) -> (-2.1187, 51.1763)
  spline S234 degree 2 poles (-2.1187, 51.1763) (-2.1187, 51.0424) (-2.2525, 51.0424) knots 0 0 0 1 1 1
  line L889 (-2.1187, 51.1763) -> (-2.1187, 51.0424) construction
  line L890 (-2.1187, 51.0424) -> (-2.2525, 51.0424) construction
  spline S235 degree 2 poles (-0.1159, 51.0424) (-0.2498, 51.0424) (-0.2498, 51.1763) knots 0 0 0 1 1 1
  line L891 (-0.1159, 51.0424) -> (-0.2498, 51.0424) construction
  line L892 (-0.2498, 51.0424) -> (-0.2498, 51.1763) construction
  line L893 (-0.2498, 51.1763) -> (-0.2498, 52.7776)
  spline S236 degree 2 poles (-0.2498, 52.7776) (-0.2498, 52.9114) (-0.1159, 52.9114) knots 0 0 0 1 1 1
  line L894 (-0.2498, 52.7776) -> (-0.2498, 52.9114) construction
  line L895 (-0.2498, 52.9114) -> (-0.1159, 52.9114) construction
  spline S237 degree 2 poles (-0.1159, 52.9114) (0.0179, 52.9114) (0.0179, 52.7776) knots 0 0 0 1 1 1
  line L896 (-0.1159, 52.9114) -> (0.0179, 52.9114) construction
  line L897 (0.0179, 52.9114) -> (0.0179, 52.7776) construction
  line L898 (0.0179, 52.7776) -> (0.0179, 51.1763)
  spline S238 degree 2 poles (0.0179, 51.1763) (0.0179, 51.0424) (-0.1159, 51.0424) knots 0 0 0 1 1 1
  line L899 (0.0179, 51.1763) -> (0.0179, 51.0424) construction
  line L900 (0.0179, 51.0424) -> (-0.1159, 51.0424) construction
  spline S239 degree 2 poles (-8.2422, 56.0349) (-8.0598, 56.0379) (-7.8015, 56.1868) (-7.7104, 56.3995) knots 0 0 0 1 2 2 2
  line L901 (-8.2422, 56.0349) -> (-8.0598, 56.0379) construction
  line L902 (-8.0598, 56.0379) -> (-7.8015, 56.1868) construction
  line L903 (-7.8015, 56.1868) -> (-7.7104, 56.3995) construction
  spline S240 degree 2 poles (-7.7104, 56.3995) (-7.683, 56.4633) (-7.6162, 56.6305) (-7.5949, 56.6943) knots 0 0 0 1 2 2 2
  line L904 (-7.7104, 56.3995) -> (-7.683, 56.4633) construction
  line L905 (-7.683, 56.4633) -> (-7.6162, 56.6305) construction
  line L906 (-7.6162, 56.6305) -> (-7.5949, 56.6943) construction
  spline S241 degree 2 poles (-7.5949, 56.6943) (-7.4855, 57.0043) (-7.0935, 57.2595) (-6.7774, 57.2595) knots 0 0 0 1 2 2 2
  line L907 (-7.5949, 56.6943) -> (-7.4855, 57.0043) construction
  line L908 (-7.4855, 57.0043) -> (-7.0935, 57.2595) construction
  line L909 (-7.0935, 57.2595) -> (-6.7774, 57.2595) construction
  spline S242 degree 2 poles (-6.7592, 56.8523) (-6.9567, 56.8523) (-7.1543, 56.6882) (-7.2211, 56.4694) knots 0 0 0 1 2 2 2
  line L910 (-6.7592, 56.8523) -> (-6.9567, 56.8523) construction
  line L911 (-6.9567, 56.8523) -> (-7.1543, 56.6882) construction
  line L912 (-7.1543, 56.6882) -> (-7.2211, 56.4694) construction
  spline S243 degree 2 poles (-7.2211, 56.4694) (-7.291, 56.2506) (-7.4825, 56.0075) (-7.5979, 55.9407) knots 0 0 0 1 2 2 2
  line L913 (-7.2211, 56.4694) -> (-7.291, 56.2506) construction
  line L914 (-7.291, 56.2506) -> (-7.4825, 56.0075) construction
  line L915 (-7.4825, 56.0075) -> (-7.5979, 55.9407) construction
  spline S244 degree 2 poles (11.9148, 54.9257) (12.0151, 54.9925) (12.1093, 55.1688) (12.1093, 55.3086) knots 0 0 0 1 2 2 2
  line L916 (11.9148, 54.9257) -> (12.0151, 54.9925) construction
  line L917 (12.0151, 54.9925) -> (12.1093, 55.1688) construction
  line L918 (12.1093, 55.1688) -> (12.1093, 55.3086) construction
  spline S245 degree 2 poles (12.1093, 55.3086) (12.1093, 55.4362) (12.0212, 55.6307) (11.9209, 55.6915) knots 0 0 0 1 2 2 2
  line L919 (12.1093, 55.3086) -> (12.1093, 55.4362) construction
  line L920 (12.1093, 55.4362) -> (12.0212, 55.6307) construction
  line L921 (12.0212, 55.6307) -> (11.9209, 55.6915) construction
  spline S246 degree 2 poles (11.9209, 55.6915) (11.8145, 55.7553) (11.5471, 55.7796) (11.2979, 55.7796) knots 0 0 0 1 2 2 2
  line L922 (11.9209, 55.6915) -> (11.8145, 55.7553) construction
  line L923 (11.8145, 55.7553) -> (11.5471, 55.7796) construction
  line L924 (11.5471, 55.7796) -> (11.2979, 55.7796) construction
  spline S247 degree 2 poles (11.2858, 54.8223) (11.538, 54.8223) (11.8145, 54.8649) (11.9148, 54.9257) knots 0 0 0 1 2 2 2
  line L925 (11.2858, 54.8223) -> (11.538, 54.8223) construction
  line L926 (11.538, 54.8223) -> (11.8145, 54.8649) construction
  line L927 (11.8145, 54.8649) -> (11.9148, 54.9257) construction
  spline S248 degree 2 poles (12.2947, 54.6765) (12.1276, 54.5519) (11.7507, 54.4455) (11.456, 54.4455) knots 0 0 0 1 2 2 2
  line L928 (12.2947, 54.6765) -> (12.1276, 54.5519) construction
  line L929 (12.1276, 54.5519) -> (11.7507, 54.4455) construction
  line L930 (11.7507, 54.4455) -> (11.456, 54.4455) construction
  spline S249 degree 2 poles (11.4681, 56.1625) (11.7842, 56.1625) (12.1336, 56.0956) (12.3068, 55.968) knots 0 0 0 1 2 2 2
  line L931 (11.4681, 56.1625) -> (11.7842, 56.1625) construction
  line L932 (11.7842, 56.1625) -> (12.1336, 56.0956) construction
  line L933 (12.1336, 56.0956) -> (12.3068, 55.968) construction
  spline S250 degree 2 poles (12.3068, 55.968) (12.4527, 55.8616) (12.5986, 55.5243) (12.5986, 55.3177) knots 0 0 0 1 2 2 2
  line L934 (12.3068, 55.968) -> (12.4527, 55.8616) construction
  line L935 (12.4527, 55.8616) -> (12.5986, 55.5243) construction
  line L936 (12.5986, 55.5243) -> (12.5986, 55.3177) construction
  spline S251 degree 2 poles (12.5986, 55.3177) (12.5986, 55.1141) (12.4345, 54.7798) (12.2947, 54.6765) knots 0 0 0 1 2 2 2
  line L937 (12.5986, 55.3177) -> (12.5986, 55.1141) construction
  line L938 (12.5986, 55.1141) -> (12.4345, 54.7798) construction
  line L939 (12.4345, 54.7798) -> (12.2947, 54.6765) construction
  spline S252 degree 2 poles (-1.6975, 14.0353) (-1.6975, 13.9009) (-1.8319, 13.9009) knots 0 0 0 1 1 1
  line L940 (-1.6975, 14.0353) -> (-1.6975, 13.9009) construction
  line L941 (-1.6975, 13.9009) -> (-1.8319, 13.9009) construction
  spline S253 degree 2 poles (-1.8319, 13.9009) (-1.9662, 13.9009) (-1.9662, 14.0353) knots 0 0 0 1 1 1
  line L942 (-1.8319, 13.9009) -> (-1.9662, 13.9009) construction
  line L943 (-1.9662, 13.9009) -> (-1.9662, 14.0353) construction
  spline S254 degree 2 poles (10.1568, 14.3355) (10.1568, 14.1499) (9.8952, 13.89) (9.7095, 13.89) knots 0 0 0 1 2 2 2
  line L944 (10.1568, 14.3355) -> (10.1568, 14.1499) construction
  line L945 (10.1568, 14.1499) -> (9.8952, 13.89) construction
  line L946 (9.8952, 13.89) -> (9.7095, 13.89) construction
  line L947 (9.7095, 13.89) -> (9.2923, 13.89)
  spline S255 degree 2 poles (9.2923, 13.89) (9.1579, 13.89) (9.1579, 14.0243) knots 0 0 0 1 1 1
  line L948 (9.2923, 13.89) -> (9.1579, 13.89) construction
  line L949 (9.1579, 13.89) -> (9.1579, 14.0243) construction
  spline S256 degree 2 poles (9.1579, 14.0243) (9.1579, 14.1569) (9.2923, 14.1569) knots 0 0 0 1 1 1
  line L950 (9.1579, 14.0243) -> (9.1579, 14.1569) construction
  line L951 (9.1579, 14.1569) -> (9.2923, 14.1569) construction
  line L952 (9.2923, 14.1569) -> (9.7095, 14.1569)
  spline S257 degree 2 poles (9.7095, 14.1569) (9.782, 14.1569) (9.8881, 14.263) (9.8881, 14.3355) knots 0 0 0 1 2 2 2
  line L953 (9.7095, 14.1569) -> (9.782, 14.1569) construction
  line L954 (9.782, 14.1569) -> (9.8881, 14.263) construction
  line L955 (9.8881, 14.263) -> (9.8881, 14.3355) construction
  spline S258 degree 2 poles (-11.8475, -26.0351) (-11.8475, -25.9013) (-11.7137, -25.9013) knots 0 0 0 1 1 1
  line L956 (-11.8475, -26.0351) -> (-11.8475, -25.9013) construction
  line L957 (-11.8475, -25.9013) -> (-11.7137, -25.9013) construction
  spline S259 degree 2 poles (-11.7137, -25.9013) (-11.5799, -25.9013) (-11.5799, -26.0351) knots 0 0 0 1 1 1
  line L958 (-11.7137, -25.9013) -> (-11.5799, -25.9013) construction
  line L959 (-11.5799, -25.9013) -> (-11.5799, -26.0351) construction
  line L960 (-11.5799, -26.0351) -> (-11.5799, -27.6364)
  spline S260 degree 2 poles (-11.5799, -27.6364) (-11.5799, -27.7703) (-11.7137, -27.7703) knots 0 0 0 1 1 1
  line L961 (-11.5799, -27.6364) -> (-11.5799, -27.7703) construction
  line L962 (-11.5799, -27.7703) -> (-11.7137, -27.7703) construction
  spline S261 degree 2 poles (-11.7137, -27.7703) (-11.8475, -27.7703) (-11.8475, -27.6364) knots 0 0 0 1 1 1
  line L963 (-11.7137, -27.7703) -> (-11.8475, -27.7703) construction
  line L964 (-11.8475, -27.7703) -> (-11.8475, -27.6364) construction
  spline S262 degree 2 poles (-12.646, -27.6364) (-12.646, -27.7703) (-12.7798, -27.7703) knots 0 0 0 1 1 1
  line L965 (-12.646, -27.6364) -> (-12.646, -27.7703) construction
  line L966 (-12.646, -27.7703) -> (-12.7798, -27.7703) construction
  spline S263 degree 2 poles (-12.7798, -27.7703) (-12.9136, -27.7703) (-12.9136, -27.6364) knots 0 0 0 1 1 1
  line L967 (-12.7798, -27.7703) -> (-12.9136, -27.7703) construction
  line L968 (-12.9136, -27.7703) -> (-12.9136, -27.6364) construction
  line L969 (-12.9136, -27.6364) -> (-12.9136, -26.0351)
  spline S264 degree 2 poles (-12.9136, -26.0351) (-12.9136, -25.9013) (-12.7798, -25.9013) knots 0 0 0 1 1 1
  line L970 (-12.9136, -26.0351) -> (-12.9136, -25.9013) construction
  line L971 (-12.9136, -25.9013) -> (-12.7798, -25.9013) construction
  spline S265 degree 2 poles (-12.7798, -25.9013) (-12.646, -25.9013) (-12.646, -26.0351) knots 0 0 0 1 1 1
  line L972 (-12.7798, -25.9013) -> (-12.646, -25.9013) construction
  line L973 (-12.646, -25.9013) -> (-12.646, -26.0351) construction
  spline S266 degree 2 poles (-6.506, -27.5026) (-6.3967, -27.5026) (-6.2406, -27.3443) (-6.2406, -27.235) knots 0 0 0 1 2 2 2
  line L974 (-6.506, -27.5026) -> (-6.3967, -27.5026) construction
  line L975 (-6.3967, -27.5026) -> (-6.2406, -27.3443) construction
  line L976 (-6.2406, -27.3443) -> (-6.2406, -27.235) construction
  line L977 (-6.2406, -27.235) -> (-6.2406, -26.4365)
  spline S267 degree 2 poles (-6.2406, -26.4365) (-6.2406, -26.3273) (-6.3967, -26.1689) (-6.506, -26.1689) knots 0 0 0 1 2 2 2
  line L978 (-6.2406, -26.4365) -> (-6.2406, -26.3273) construction
  line L979 (-6.2406, -26.3273) -> (-6.3967, -26.1689) construction
  line L980 (-6.3967, -26.1689) -> (-6.506, -26.1689) construction
  spline S268 degree 2 poles (-7.039, -28.4371) (-7.039, -28.5709) (-7.1728, -28.5709) knots 0 0 0 1 1 1
  line L981 (-7.039, -28.4371) -> (-7.039, -28.5709) construction
  line L982 (-7.039, -28.5709) -> (-7.1728, -28.5709) construction
  spline S269 degree 2 poles (-7.1728, -28.5709) (-7.3067, -28.5709) (-7.3067, -28.4371) knots 0 0 0 1 1 1
  line L983 (-7.1728, -28.5709) -> (-7.3067, -28.5709) construction
  line L984 (-7.3067, -28.5709) -> (-7.3067, -28.4371) construction
  line L985 (-7.3067, -28.4371) -> (-7.3067, -26.0351)
  spline S270 degree 2 poles (-7.3067, -26.0351) (-7.3067, -25.9013) (-7.1728, -25.9013) knots 0 0 0 1 1 1
  line L986 (-7.3067, -26.0351) -> (-7.3067, -25.9013) construction
  line L987 (-7.3067, -25.9013) -> (-7.1728, -25.9013) construction
  line L988 (-7.1728, -25.9013) -> (-6.506, -25.9013)
  spline S271 degree 2 poles (-6.506, -25.9013) (-6.2852, -25.9013) (-5.973, -26.2135) (-5.973, -26.4343) knots 0 0 0 1 2 2 2
  line L989 (-6.506, -25.9013) -> (-6.2852, -25.9013) construction
  line L990 (-6.2852, -25.9013) -> (-5.973, -26.2135) construction
  line L991 (-5.973, -26.2135) -> (-5.973, -26.4343) construction
  line L992 (-5.973, -26.4343) -> (-5.973, -27.2372)
  spline S272 degree 2 poles (-5.973, -27.2372) (-5.973, -27.458) (-6.2852, -27.7703) (-6.506, -27.7703) knots 0 0 0 1 2 2 2
  line L993 (-5.973, -27.2372) -> (-5.973, -27.458) construction
  line L994 (-5.973, -27.458) -> (-6.2852, -27.7703) construction
  line L995 (-6.2852, -27.7703) -> (-6.506, -27.7703) construction
  spline S273 degree 2 poles (-4.637, -27.5026) (-4.5277, -27.5026) (-4.3716, -27.3443) (-4.3716, -27.235) knots 0 0 0 1 2 2 2
  line L996 (-4.637, -27.5026) -> (-4.5277, -27.5026) construction
  line L997 (-4.5277, -27.5026) -> (-4.3716, -27.3443) construction
  line L998 (-4.3716, -27.3443) -> (-4.3716, -27.235) construction
  spline S274 degree 2 poles (-4.9046, -26.1689) (-5.0139, -26.1689) (-5.1701, -26.3273) (-5.1701, -26.4365) knots 0 0 0 1 2 2 2
  line L999 (-4.9046, -26.1689) -> (-5.0139, -26.1689) construction
  line L1000 (-5.0139, -26.1689) -> (-5.1701, -26.3273) construction
  line L1001 (-5.1701, -26.3273) -> (-5.1701, -26.4365) construction
  line L1002 (-5.1701, -26.4365) -> (-5.1701, -27.235)
  spline S275 degree 2 poles (-5.1701, -27.235) (-5.1701, -27.3443) (-5.0139, -27.5026) (-4.9046, -27.5026) knots 0 0 0 1 2 2 2
  line L1003 (-5.1701, -27.235) -> (-5.1701, -27.3443) construction
  line L1004 (-5.1701, -27.3443) -> (-5.0139, -27.5026) construction
  line L1005 (-5.0139, -27.5026) -> (-4.9046, -27.5026) construction
  line L1006 (-4.9046, -27.5026) -> (-4.637, -27.5026)
  line L1007 (-4.637, -27.7703) -> (-4.9046, -27.7703)
  spline S276 degree 2 poles (-4.9046, -27.7703) (-5.1232, -27.7703) (-5.4377, -27.458) (-5.4377, -27.2372) knots 0 0 0 1 2 2 2
  line L1008 (-4.9046, -27.7703) -> (-5.1232, -27.7703) construction
  line L1009 (-5.1232, -27.7703) -> (-5.4377, -27.458) construction
  line L1010 (-5.4377, -27.458) -> (-5.4377, -27.2372) construction
  line L1011 (-5.4377, -27.2372) -> (-5.4377, -26.4343)
  spline S277 degree 2 poles (-5.4377, -26.4343) (-5.4377, -26.2135) (-5.1232, -25.9013) (-4.9046, -25.9013) knots 0 0 0 1 2 2 2
  line L1012 (-5.4377, -26.4343) -> (-5.4377, -26.2135) construction
  line L1013 (-5.4377, -26.2135) -> (-5.1232, -25.9013) construction
  line L1014 (-5.1232, -25.9013) -> (-4.9046, -25.9013) construction
  line L1015 (-4.9046, -25.9013) -> (-4.2378, -25.9013)
  spline S278 degree 2 poles (-4.2378, -25.9013) (-4.104, -25.9013) (-4.104, -26.0351) knots 0 0 0 1 1 1
  line L1016 (-4.2378, -25.9013) -> (-4.104, -25.9013) construction
  line L1017 (-4.104, -25.9013) -> (-4.104, -26.0351) construction
  line L1018 (-4.104, -26.0351) -> (-4.104, -27.2328)
  spline S279 degree 2 poles (-4.104, -27.2328) (-4.104, -27.4335) (-3.9166, -27.5138) knots 0 0 0 1 1 1
  line L1019 (-4.104, -27.2328) -> (-4.104, -27.4335) construction
  line L1020 (-4.104, -27.4335) -> (-3.9166, -27.5138) construction
  spline S280 degree 2 poles (-3.9166, -27.5138) (-3.8341, -27.5472) (-3.8341, -27.632) knots 0 0 0 1 1 1
  line L1021 (-3.9166, -27.5138) -> (-3.8341, -27.5472) construction
  line L1022 (-3.8341, -27.5472) -> (-3.8341, -27.632) construction
  spline S281 degree 2 poles (-3.8341, -27.632) (-3.8341, -27.6877) (-3.9099, -27.7725) (-3.9657, -27.7725) knots 0 0 0 1 2 2 2
  line L1023 (-3.8341, -27.632) -> (-3.8341, -27.6877) construction
  line L1024 (-3.8341, -27.6877) -> (-3.9099, -27.7725) construction
  line L1025 (-3.9099, -27.7725) -> (-3.9657, -27.7725) construction
  spline S282 degree 2 poles (-3.9657, -27.7725) (-3.9947, -27.7725) (-4.0237, -27.7591) knots 0 0 0 1 1 1
  line L1026 (-3.9657, -27.7725) -> (-3.9947, -27.7725) construction
  line L1027 (-3.9947, -27.7725) -> (-4.0237, -27.7591) construction
  spline S283 degree 2 poles (-4.0237, -27.7591) (-4.1575, -27.7011) (-4.24, -27.5941) knots 0 0 0 1 1 1
  line L1028 (-4.0237, -27.7591) -> (-4.1575, -27.7011) construction
  line L1029 (-4.1575, -27.7011) -> (-4.24, -27.5941) construction
  spline S284 degree 2 poles (-4.24, -27.5941) (-4.4006, -27.7703) (-4.637, -27.7703) knots 0 0 0 1 1 1
  line L1030 (-4.24, -27.5941) -> (-4.4006, -27.7703) construction
  line L1031 (-4.4006, -27.7703) -> (-4.637, -27.7703) construction
  line L1032 (-3.3011, -25.5801) -> (-3.3011, -25.9949)